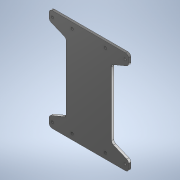
# Autodesk Inventor part: Controller - Power Board v2
Saved by Autodesk Inventor 2020.2 (Build 242310000, 310)
## iProperties
Created: 2020-08-26
Part Number: Controller - Power Board v2
Material: Generic
Document SubType Name: Modeling
Designer: Krishna Makhija
Density: 1 g/cm^3
Appearance: Default
Author: Krishna Makhija
Autodesk Inventor part; units mm, degrees
ref_plane "YZ Plane" through (0, 0, 0) normal (1, 0, 0) x (0, 1, 0)
ref_plane "XZ Plane" through (0, 0, 0) normal (0, 1, 0) x (-1, 0, 0)
ref_plane "XY Plane" through (0, 0, 0) normal (0, 0, 1) x (1, 0, 0)
sketch "Sketch1" plane through (0, 0, 0) normal (0, 0, 1) x (1, 0, 0)
  point P0 (0, 0)
sketch "Sketch2" plane through (0, 0, 0) normal (0, 0, 1) x (1, 0, 0)
  line L0 (-52.4998, -67.5002) -> (52.4998, -67.5002)
  line L1 (52.4998, -67.5002) -> (52.4998, 67.5002)
  line L2 (52.4998, 67.5002) -> (-52.4998, 67.5002)
  line L3 (-52.4998, 67.5002) -> (-52.4998, -67.5002)
  circle A0 centre (48, 60) radius 1.5002
  circle A1 centre (-48, 60) radius 1.5002
  circle A2 centre (-48, -60) radius 1.5002
  circle A3 centre (48, -60) radius 1.5002
  circle A4 centre (22, 60) radius 1.4999
  circle A5 centre (-22, 60) radius 1.4999
  circle A6 centre (22, -60) radius 1.4999
  circle A7 centre (-22, -60) radius 1.4999
  line L4 (0, -44.9999) -> (0, 44.9999)
  line L5 (30, -44.9999) -> (30, 44.9999)
  line L6 (30, 44.9999) -> (52.4998, 54.3179)
  line L7 (30, -44.9999) -> (52.4998, -54.3208)
  line L8 (-30, -44.9999) -> (-30, 44.9999)
  line L9 (-30, 44.9999) -> (-52.4998, 54.3179)
  line L10 (-30, -44.9999) -> (-52.4998, -54.3208)
  constraints: 22 end point, 8 centre point, 4 coincident, 4 symmetric about line, 2 parallel, 2 point on line, 2 vertical, 1 horizontal, 1 perpendicular
extrude "Extrusion3" add sketch "Sketch2" along normal blind 3
fillet "Fillet4" radius 4 4 edges at (-52.4998, 67.5002, 1.5) (52.4998, 67.5002, 1.5) (52.4998, -67.5002, 1.5) (-52.4998, -67.5002, 1.5)
extrude "Extrusion4" cut sketch "Sketch2" along normal blind 10 contours L3 L9 L8 L10 | L7 L5 L6 L1
fillet "Fillet5" radius 4 8 edges at (52.4998, 54.3179, 1.5) (30, 44.9999, 1.5) (-30, 44.9999, 1.5) (-52.4998, 54.3179, 1.5) (-30, -44.9999, 1.5) (-52.4998, -54.3208, 1.5) (30, -44.9999, 1.5) (52.4998, -54.3208, 1.5)
body "Solid2"
